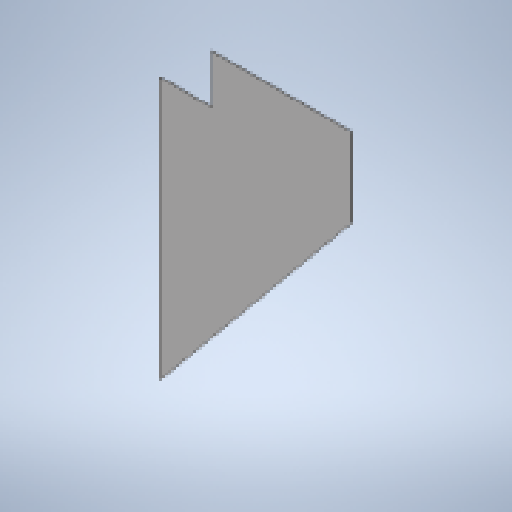
# Autodesk Inventor part: МОО 052 гребень 2
Saved by Autodesk Inventor 2024.2 (Build 282272000, 272)
## iProperties
Created: 2024-06-08
Part Number: МОО 052 гребень 2
Material: Generic
Document SubType Name: Sheet Metal
Designer: admin
Density: 1 g/cm^3
Sheet Metal Rule: Default
Appearance: Default
Author: admin
Autodesk Inventor part; units mm, degrees
ref_plane "YZ Plane" through (0, 0, 0) normal (1, 0, 0) x (0, 1, 0)
ref_plane "XZ Plane" through (0, 0, 0) normal (0, 1, 0) x (-1, 0, 0)
ref_plane "XY Plane" through (0, 0, 0) normal (0, 0, 1) x (1, 0, 0)
sketch "Sketch1" plane through (0, 0, 0) normal (0, 1, 0) x (-1, 0, 0)
  line L0 (-750.7615, 0) -> (-750.7615, -1064.7696)
  line L1 (-750.7615, -1064.7696) -> (-100, -1741.0083)
  line L2 (0, -1741.0083) -> (0, 0)
  line L3 (0, 0) -> (-750.7615, 0)
  line L4 (0, -200) -> (-213.3206, -200)
  line L5 (-213.3206, -200) -> (-213.3206, 0)
  line L6 (-100, -1741.0083) -> (0, -1741.0083)
  dimension "d0" = 1064.77
  dimension "d2" = 1741.008
  dimension "d5" = 200
  dimension "d6" = 213.3206
  dimension "d7" = 1741.008
  dimension "d8" = 100
  measures "d0" distance of L0.start L0.end
  measures "d2" distance of L2.start L2.end
  measures "d5" distance between parallel lines of L3 L4
  measures "d6" distance between parallel lines of L2 L5
  measures "d7" distance between parallel lines of L3 L6
  measures "d8" distance of L1.end L2.start
extrude "Plate1" add sketch "Sketch1" along normal blind 2 contours L3 L5 L4 L2 L6 L1 L0
equation "\"d3\" = Thickness"
equation "\"BendRadius\" = Thickness"
equation "\"BendReliefWidth\" = Thickness"
equation "\"BendReliefDepth\" = 0.5 * Thickness"
equation "\"CornerReliefSize\" = 4 * Thickness"
equation "\"MinimumRemnant\" = 2 * Thickness"
equation "\"TransitionRadius\" = BendRadius"
equation "\"JacobiRadiusSize\" = BendRadius"
equation "\"GapSize\" = Thickness"
equation "\"Thickness\" = 2"
body "Solid1"
